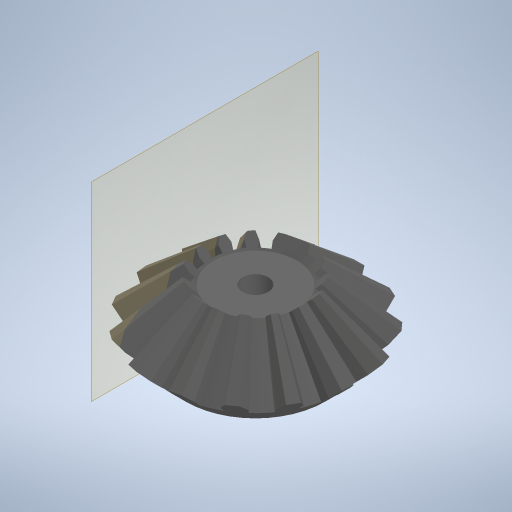
# Autodesk Inventor part: M3_15_crown_in
Saved by Autodesk Inventor 2024.1 (Build 281209000, 209)
## iProperties
Created: 2024-04-01
Part Number: M3_15_crown_in
Material: 一般
Document SubType Name: Modeling
Designer: hibik
Density: 1 g/cm^3
Appearance: 既定
Author: hibik
Autodesk Inventor part; units mm, degrees
ref_plane "XZ Plane" through (0, 0, 0) normal (0, 1, 0) x (-1, 0, 0)
ref_plane "XY Plane" through (0, 0, 0) normal (0, 0, 1) x (1, 0, 0)
sketch "スケッチ3" plane through (0, 0, 0) normal (1, 0, 0) x (0, 1, 0)
  line L0 (0, 0) -> (-20, -24.2426)
  line L1 (0, 0) -> (-24.773, -19.4697)
  line L2 (0, 0) -> (-33.8756, -33.8756) construction
  line L3 (-24.773, -19.4697) -> (-20, -24.2426)
  line L4 (-10, -12.1213) -> (-12.3865, -9.7348)
  line L5 (-40.6507, 0) -> (6.7751, 0) projected
  line L6 (-24.773, -19.4697) -> (-28, -16.2426)
  line L7 (-28, -16.2426) -> (-28, 0)
  line L8 (-12.3865, -9.7348) -> (-12.3865, 0)
  line L9 (-12.0304, -10.0909) -> (-24.4169, -19.8258)
  dimension "d28" = 45
  dimension "d29" = 3.75
  dimension "d30" = 3
  dimension "d31" = 20
  dimension "d32" = 10
  dimension "d33" = 28
  dimension "d66" = 0.5
  constraints: 18 end point, 7 point on line, 3 midpoint, 3 perpendicular, 2 parallel, 1 collinear
  measures "d28" angle of L5 L2
  measures "d29" distance from line of L3.start L2
  measures "d30" distance from line of L3.end L2
  measures "d31" horizontal distance of L0.start L3.end
  measures "d32" horizontal distance of L0.start L4.start
  measures "d33" distance from line of L7 L0.start
  measures "d66" distance between parallel lines of L9 L1
extrude "押し出し3" add sketch "スケッチ3" along normal mid plane 10 contours L0 L3 L9 L4 | L4 L9 L3 L1
sketch "スケッチ4" plane through (5, -20, -24.2426) normal (0, -0.7071068, -0.7071068) x (-1, 0, 0)
  line L0 (5, 1.4202) -> (5, -6.75) construction
  line L1 (0, 0) -> (10, 0) projected
  line L2 (3.7369, 0) -> (2.645, -3)
  line L3 (2.645, -3) -> (3.038, -6.75)
  line L4 (6.962, -6.75) -> (7.355, -3)
  line L5 (7.355, -3) -> (6.2631, 0)
  circle A0 centre (5, -25.4687) radius 25.5 construction
  line L6 (0, 0) -> (10, 0) projected
  line L7 (0, -6.75) -> (0, 0) construction
  line L8 (10, -6.75) -> (0, -6.75) projected
  line L9 (10, 0) -> (10, -6.75) construction
  line L10 (6.962, -6.75) -> (5, -25.4687) construction
  line L11 (5, -25.4687) -> (5, -6.75) construction
  line L12 (3.038, -6.75) -> (5, -25.4687) construction
  point P0 (5, -3)
  point P1 (3.038, -6.75)
  dimension "d36" = 51
  dimension "d37" = 20
  dimension "d42" = 4.71
  dimension "d43" = 3
  constraints: 16 end point, 5 point on line, 2 vertical, 1 collinear, 1 midpoint, 5 other
  measures "d37" angle of L0 L2
  measures "d42" distance of L4.end L2.end
  measures "d43" distance from line of L2.end L1
sketch "スケッチ7" plane through (-5, -12.3865, -9.7348) normal (0, 0.7071068, 0.7071068) x (1, 0, 0)
  line L0 (10, 4.875) -> (0, 4.875) construction
  line L1 (10, -1.875) -> (10, 4.875) construction
  line L2 (0, -1.875) -> (10, -1.875) construction
  line L3 (0, 4.875) -> (0, -1.875) construction
  line L4 (0, 1.875) -> (10, 1.875) construction
  line L5 (4.3685, 3.375) -> (3.8225, 1.875)
  line L6 (4.0494, 0) -> (3.8225, 1.875)
  line L7 (5, -7.8573) -> (5, 3.3151) construction
  line L8 (5.6315, 3.375) -> (6.1775, 1.875)
  line L9 (5.9506, 0) -> (6.1775, 1.875)
  line L10 (4.2762, -1.875) -> (5, -7.8573) construction
  line L11 (5.7238, -1.875) -> (5, -7.8573) construction
  line L12 (0, 0) -> (10, 0) projected
  line L13 (0, 3.375) -> (10, 3.375) projected
  circle A0 centre (5, -7.8573) radius 11.25 construction
  line L14 (4.0494, 0) -> (5.9506, 0)
  line L15 (6.1775, 1.875) -> (5.6315, 3.375)
  line L16 (4.3685, 3.375) -> (5.6315, 3.375)
  line L17 (4.3685, 3.375) -> (3.8225, 1.875)
  line L18 (3.8225, 1.875) -> (4.0494, 0)
  line L19 (5.9506, 0) -> (6.1775, 1.875)
  point P0 (5, 1.875)
  point P1 (5, 1.875)
  dimension "d55" = 22.5
  dimension "d51" = 3
  dimension "d52" = 20
  dimension "d53" = 2.355
  dimension "d54" = 3.375
  constraints: 28 end point, 9 point on line, 5 collinear, 2 symmetric about line, 1 coincident, 1 horizontal, 1 midpoint, 1 vertical, 3 other
  measures "d51" distance between parallel lines of L0 L4
  measures "d52" angle of L7 L5
  measures "d53" distance of L8.end L5.end
  measures "d54" distance between parallel lines of L12 L13
sketch "スケッチ8" plane through (5, -20, -24.2426) normal (0, -0.7071068, -0.7071068) x (-1, 0, 0)
  line L0 (0, 0) -> (10, 0) projected
  line L1 (0, -6.75) -> (0, 0) projected
  line L2 (10, -6.75) -> (0, -6.75) projected
  line L3 (10, 0) -> (10, -6.75) projected
  point P0 (5, -3)
extrude "押し出し6" cut sketch "スケッチ8" against normal through all
loft "ロフト1" add profiles "スケッチ4", "スケッチ7"
pattern_circular "円形状パターン1" count 15 over 360 about axis through (0, -10, 0) along (0, 1, 0)
revolve "回転1" add sketch "スケッチ3" angle 360 about axis through (0, -10, 0) along (0, 1, 0) contours L4 L9 L3 L1 | L1 L6 L7 L5 L8
sketch "スケッチ10" plane through (0, -12.3865, 0) normal (0, 1, 0) x (1, 0, 0)
  circle A0 centre (0, 0) radius 3
  dimension "d71" = 6
  constraints: 1 centre point, 1 coincident
  measures "d71" diameter of A0
extrude "押し出し8" cut sketch "スケッチ10" against normal through all
sketch "スケッチ12" plane through (0, 0, 0) normal (1, 0, 0) x (0, 1, 0)
  circle A0 centre (-25, 0) radius 1.25
  point P0 (0, 0)
  dimension "d75" = 2.5
  dimension "d76" = 25
  constraints: 1 centre point, 1 horizontal alignment
  measures "d75" diameter of A0
  measures "d76" distance of point (0, 0) A0.centre
extrude "押し出し9" cut sketch "スケッチ12" against normal through all
ref_plane "作業平面2" through (-12, 0, 0) normal (1, 0, 0) x (0, 1, 0)
sketch "スケッチ13" plane through (-12, 0, 0) normal (1, 0, 0) x (0, 1, 0)
  arc A0 (-23.7506, 0.0401) -> (-24.773, 1.2292) centre (-25, 0) ccw projected
  circle A1 centre (-25, 0) radius 3
  point P0 (0, 0)
  dimension "d80" = 6
  constraints: 1 centre point, 1 coincident, 2 other
  measures "d80" diameter of A1
extrude "押し出し10" cut sketch "スケッチ13" against normal through all
equation "\"d55\" = 6.66667 * d54"
equation "\"d53\" = 0.697778 * d54"
